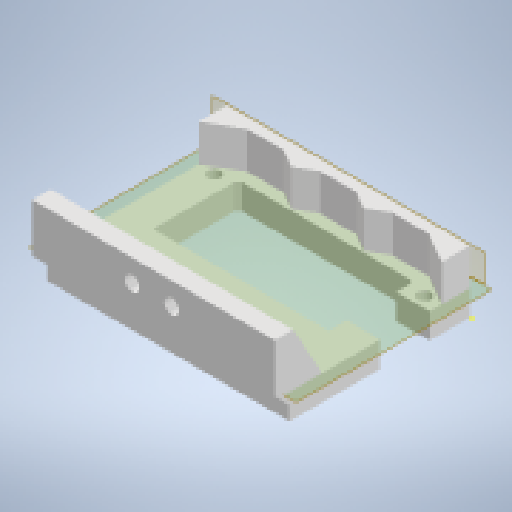
# Autodesk Inventor part: делать держит аккум
Saved by Autodesk Inventor 2024.2 (Build 282272000, 272)
## iProperties
Created: 2026-04-23
Part Number: делать держит аккум
Material: Типовые
Document SubType Name: Sheet Metal
Designer: katya_notebook
Density: 1 g/cm^3
Appearance: По умолчанию
Sheet Metal Rule: По умолчанию
Author: katya_notebook
Autodesk Inventor part; units mm, degrees
(part 1 of 2)
ref_plane "YZ Plane" through (0, 0, 0) normal (1, 0, 0) x (0, 1, 0)
ref_plane "XZ Plane" through (0, 0, 0) normal (0, 1, 0) x (-1, 0, 0)
ref_plane "XY Plane" through (0, 0, 0) normal (0, 0, 1) x (1, 0, 0)
ref_plane "РабПлоскость1" through (0, 0, 0) normal (0, 0, 1) x (1, 0, 0)
sketch "Эскиз1" plane through (0, 0, 0) normal (0, 0, 1) x (1, 0, 0)
  line L0 (-67, 0) -> (-67, 6.8113) projected
  line L1 (-67, 6.8113) -> (-59, 6.8113)
  line L2 (-59, 6.8113) -> (-59, 0)
  line L3 (-59, 0) -> (-67, 0)
  line L4 (-67, 0) -> (-67, 6.8113)
  line L5 (0, 6.8113) -> (0, 0) projected
  line L6 (0, 0) -> (-8, 0)
  line L7 (-8, 0) -> (-8, 6.8113)
  line L8 (-8, 6.8113) -> (0, 6.8113)
  line L9 (0, 6.8113) -> (0, 0)
  circle A0 centre (-62.5001, 3.4873) radius 2.1 projected
  circle A1 centre (-4.4999, 3.4873) radius 2.1 projected
  dimension "d0" = 8
  dimension "d1" = 8
  constraints: 16 end point, 4 parallel, 2 horizontal, 2 perpendicular
  measures "d0" distance of L0.end L1.end
  measures "d1" distance of L7.end L8.end
extrude "Выдавливание1" add sketch "Эскиз1" along normal blind 3
sketch "Эскиз2" plane through (-8, 0, 0) normal (0, -1, 0) x (1, 0, 0)
  line L0 (-49.3908, 28.0506) -> (-48.3929, 29.0527) projected
  line L1 (-48.3929, 29.0527) -> (-2.693, 29.1496) projected
  line L2 (-2.693, 29.1496) -> (-1.6909, 28.1517) projected
  line L3 (-1.6909, 28.1517) -> (-1.6464, 7.1518) projected
  line L4 (-1.6464, 7.1518) -> (-2.6442, 6.1496) projected
  line L5 (-2.6442, 6.1496) -> (-48.3441, 6.0528) projected
  line L6 (-48.3441, 6.0528) -> (-49.3463, 7.0507) projected
  line L7 (-49.3463, 7.0507) -> (-49.3908, 28.0506) projected
  line L8 (-48.6136, 30.0985) -> (-51.1395, 27.2282) projected
  line L9 (-51.1395, 27.2282) -> (-54.9179, 25.0466) projected
  line L10 (-54.9179, 25.0466) -> (-58.4036, 23.0363) projected
  line L11 (-58.4036, 23.0363) -> (-58.4, 21.3316) projected
  line L12 (-58.4, 21.3316) -> (-58.4, 9.3834) projected
  line L13 (-58.4, 9.3834) -> (-58.3964, 7.6788) projected
  line L14 (-58.3964, 7.6788) -> (-54.9179, 5.6684) projected
  line L15 (-54.9179, 5.6684) -> (-45.1, 0) projected
  line L16 (-45.1, 0) -> (-35.296, 5.6604) projected
  line L17 (-35.296, 5.6604) -> (-25.4498, 0.0035) projected
  line L18 (-25.4498, 0.0035) -> (-22.0179, 2.0104) projected
  line L19 (-22.0179, 2.0104) -> (-15.7, 5.658) projected
  line L20 (-15.7, 5.658) -> (-5.9, 0) projected
  line L21 (-5.9, 0) -> (3.9179, 5.6684) projected
  line L22 (3.9179, 5.6684) -> (7.4036, 7.6788) projected
  line L23 (7.4036, 7.6788) -> (7.4, 9.3834) projected
  line L24 (7.4, 9.3834) -> (7.4, 21.3316) projected
  line L25 (7.4, 21.3316) -> (7.3964, 23.0363) projected
  line L26 (7.3964, 23.0363) -> (3.9179, 25.0466) projected
  line L27 (3.9179, 25.0466) -> (-0.048, 27.3364) projected
  line L28 (-0.048, 27.3364) -> (-2.4, 30.1965) projected
  line L29 (-2.4, 30.1965) -> (-2.4, 38.3057) projected
  line L30 (-2.4, 38.3057) -> (-2.4036, 40.0104) projected
  line L31 (-2.4036, 40.0104) -> (-5.8821, 42.0207) projected
  line L32 (-5.8821, 42.0207) -> (-15.7, 47.6891) projected
  line L33 (-15.7, 47.6891) -> (-15.7258, 47.6742) projected
  line L34 (-15.7258, 47.6742) -> (-15.7517, 47.6891) projected
  line L35 (-15.7517, 47.6891) -> (-35.3517, 47.6891) projected
  line L36 (-35.3517, 47.6891) -> (-48.6347, 40.0202) projected
  line L37 (-48.6347, 40.0202) -> (-48.6136, 30.0985) projected
  line L38 (8, 0) -> (8, 3) projected
  line L39 (0, 0) -> (0, 3) projected
  line L40 (-51, 0) -> (-51, 3) projected
  line L41 (-59, 0) -> (-59, 3) projected
  line L42 (8, 3) -> (8, 8.0252)
  line L43 (8, 8.0252) -> (8, 8.0252)
  line L44 (-59, 3) -> (-51, 3) projected
  line L45 (-51, 3) -> (-51, 3.4064)
  line L46 (-59, 3) -> (-59, 8.0252)
  line L47 (-59, 8.0252) -> (-51, 3.4064)
  line L48 (0, 3) -> (0, 3.4064)
  line L49 (8, 8.0252) -> (0, 3.4064)
  line L50 (0, 3) -> (8, 3) projected
  line L51 (0, 0) -> (-51, 0)
  line L52 (1.4001, 3) -> (1.4001, 0) projected
  circle A0 centre (-54, 8) radius 2.1 projected
  circle A1 centre (3, 8) radius 2.1 projected
  point P0 (7.4036, 7.6808)
  point P1 (-5.9, 0)
  point P2 (-5.9, 0)
  point P3 (-45.1, 0)
  point P4 (-45.1, 0)
  constraints: 16 end point, 4 point on line, 2 parallel, 2 vertical, 1 collinear, 1 perpendicular
extrude "Выдавливание2" add sketch "Эскиз2" against normal up to surface (6.8113 mm away) contours L14 L15 L45 L44 L46 L47 | L15 L51 L40 L45 | L16 L17 L18 L19 L20 L51 | L21 L48 L39 L51 | L21 L22 L49 L42 L50 L48
sketch "Эскиз3" plane through (-13.9, 0, 0) normal (0, -1, 0) x (1, 0, 0)
  line L0 (0, 0) -> (13.9, 0) projected
  line L1 (13.9, 0) -> (13.9, 8.0252) projected
  line L2 (13.9, 8.0252) -> (13.3036, 7.6808) projected
  line L3 (13.3036, 7.6808) -> (13.3036, 7.6788) projected
  line L4 (13.3036, 7.6788) -> (9.8179, 5.6684) projected
  line L5 (9.8179, 5.6684) -> (0, 0) projected
  line L6 (-16.1179, 2.0104) -> (-19.5498, 0.0035) projected
  line L7 (-19.5498, 0.0035) -> (-29.396, 5.6604) projected
  line L8 (-29.396, 5.6604) -> (-39.2, 0) projected
  line L9 (-39.2, 0) -> (0, 0) projected
  line L10 (0, 0) -> (-9.8, 5.658) projected
  line L11 (-9.8, 5.658) -> (-16.1179, 2.0104) projected
  line L12 (-53.1, 0) -> (-39.2, 0) projected
  line L13 (-39.2, 0) -> (-53.1, 8.0252) projected
  line L14 (-53.1, 0) -> (-53.1, 8.0252) projected
  point P0 (13.9, 0)
ref_plane "РабПлоскость2" through (-66.4944, -3.1253, -0.1297) normal (0, -1, 0) x (0.9999978, 0, 0.0021189)
extrude "Выдавливание3" add sketch "Эскиз3" along normal blind 10
ref_plane "РабПлоскость3" through (-33.518, -3.1253, 23.8341) normal (0, -1, 0) x (0.9999978, 0, 0.0021189)
sketch "Эскиз4" plane through (-33.518, -3.1253, 23.8341) normal (0, -1, 0) x (0.9999978, 0, 0.0021189)
  line L0 (-23.8638, 4.267) -> (-22.8638, 5.267) projected
  line L1 (-22.8638, 5.267) -> (22.8362, 5.2671) projected
  line L2 (22.8362, 5.2671) -> (23.8362, 4.2671) projected
  line L3 (23.8362, 4.2671) -> (23.8362, -16.7329) projected
  line L4 (23.8362, -16.7329) -> (22.8362, -17.7329) projected
  line L5 (22.8362, -17.7329) -> (-22.8638, -17.733) projected
  line L6 (-22.8638, -17.733) -> (-23.8638, -16.733) projected
  line L7 (-23.8638, -16.733) -> (-23.8638, 4.267) projected
  line L8 (-23.0824, 6.3133) -> (-25.6142, 3.4483) projected
  line L9 (-25.6142, 3.4483) -> (-29.3974, 1.2748) projected
  line L10 (-29.3974, 1.2748) -> (-32.8873, -0.7282) projected
  line L11 (-32.8873, -0.7282) -> (-32.8873, -2.4329) projected
  line L12 (-32.8873, -2.4329) -> (-32.9126, -14.381) projected
  line L13 (-32.9126, -14.381) -> (-32.9126, -16.0857) projected
  line L14 (-32.9126, -16.0857) -> (-29.4384, -18.1034) projected
  line L15 (-29.4384, -18.1034) -> (-19.6325, -23.7926) projected
  line L16 (-19.6325, -23.7926) -> (-9.8165, -18.153) projected
  line L17 (-9.8165, -18.153) -> (0.0176, -23.8308) projected
  line L18 (0.0176, -23.8308) -> (3.4538, -21.8311) projected
  line L19 (3.4538, -21.8311) -> (9.7794, -18.1969) projected
  line L20 (9.7794, -18.1969) -> (19.5674, -23.8757) projected
  line L21 (19.5674, -23.8757) -> (29.3974, -18.2281) projected
  line L22 (29.3974, -18.2281) -> (32.8873, -16.2251) projected
  line L23 (32.8873, -16.2251) -> (32.8873, -14.5204) projected
  line L24 (32.8873, -14.5204) -> (32.9126, -2.5723) projected
  line L25 (32.9126, -2.5723) -> (32.9126, -0.8676) projected
  line L26 (32.9126, -0.8676) -> (29.4384, 1.1501) projected
  line L27 (29.4384, 1.1501) -> (25.4773, 3.4483) projected
  line L28 (25.4773, 3.4483) -> (23.1314, 6.3133) projected
  line L29 (23.1314, 6.3133) -> (23.1486, 14.4226) projected
  line L30 (23.1486, 14.4226) -> (23.1486, 16.1272) projected
  line L31 (23.1486, 16.1272) -> (19.6744, 18.1449) projected
  line L32 (19.6744, 18.1449) -> (9.8685, 23.8341) projected
  line L33 (9.8685, 23.8341) -> (9.8426, 23.8193) projected
  line L34 (9.8426, 23.8193) -> (9.8168, 23.8342) projected
  line L35 (9.8168, 23.8342) -> (-9.7831, 23.8758) projected
  line L36 (-9.7831, 23.8758) -> (-23.0824, 16.235) projected
  line L37 (-23.0824, 16.235) -> (-23.0824, 6.3133) projected
  line L38 (32.8916, -12.4579) -> (23.8362, -12.4579)
  line L39 (-23.8638, -12.4579) -> (-32.9085, -12.4579)
  circle A0 centre (-28.5155, -15.7738) radius 2.1 projected
  circle A1 centre (28.4843, -15.8945) radius 2.1 projected
  point P0 (33.4674, -23.9051)
  constraints: 6 point on line, 4 end point, 1 perpendicular
extrude "Выдавливание4" add sketch "Эскиз4" along normal up to surface (6.8747 mm away) contours L7 L6 L5 L4 L3 L38 L24 L23 L22 L21 L20 L19 L18 L17 L16 L15 L14 L13 L12 L39 | A0 | A1
sketch "Эскиз6" plane through (-67, 6.8113, 0) normal (0, 1, 0) x (1, 0, 0)
  line L0 (62.9179, -5.6684) -> (53.1, 0) projected
  line L1 (58.009, -2.8342) -> (0, -2.8342)
  line L2 (0, 0) -> (0, -8.0252) projected
  line L3 (58.009, -2.8342) -> (67, -2.8342)
  line L4 (67, -2.8342) -> (67, 0)
  line L5 (67, 0) -> (0, 0)
  constraints: 8 end point, 2 perpendicular, 2 point on line, 1 horizontal, 1 midpoint
ref_plane "РабПлоскость4" through (-66.4944, 1.8747, -0.1297) normal (0, 1, 0) x (-0.0021189, 0, 0.9999978)
extrude "Выдавливание6" add sketch "Эскиз6" against normal blind 12.687
sketch "Эскиз5" plane through (-13.9, -10, 0) normal (0, -1, 0) x (1, 0, 0)
  circle A0 centre (8.9, 8) radius 1.75
  line L0 (13.9, 0) -> (13.9, 8.0252) projected
  line L1 (-53.1, 0) -> (13.9, 0) projected
  circle A1 centre (-48.1, 8) radius 1.75
  line L2 (-53.1, 8.0252) -> (-53.1, 0) projected
  dimension "d10" = 3.5
  dimension "d11" = 5
  dimension "d12" = 8
  dimension "d13" = 5
  dimension "d14" = 8
  constraints: 2 centre point, 1 equal radius
  measures "d10" diameter of A0
  measures "d11" distance from line of L0 A0.centre
  measures "d12" distance from line of L1 A0.centre
  measures "d13" distance from line of L2 A1.centre
  measures "d14" distance from line of L1 A1.centre
extrude "Выдавливание5" cut sketch "Эскиз5" against normal blind 20
sketch "Эскиз7" plane through (-57.3553, -10, 11.3257) normal (-0.0021195, 0, 0.9999978) x (0.9999978, 0, 0.0021195)
  line L0 (-9.0447, 0) -> (0, 0) projected
  line L1 (0, 6.8747) -> (0, 0) projected
  line L2 (0, 6.8747) -> (-9.0447, 6.8747) projected
  line L3 (-9.0447, 6.8747) -> (-9.0447, 0) projected
  line L4 (47.7, 0) -> (56.7554, 0) projected
  line L5 (56.7554, 6.8747) -> (56.7554, 0) projected
  line L6 (56.7554, 6.8747) -> (47.7, 6.8747) projected
  line L7 (47.7, 6.8747) -> (47.7, 0) projected
  point P0 (57.3312, 10)
ref_plane "РабПлоскость5" through (-43.3847, -3.2558, 47.6891) normal (0, 0, 1) x (1, 0, 0)
extrude "Выдавливание7" add sketch "Эскиз7" along normal up to surface surface through (-43.3847, -3.2558, 47.6891) normal (0, 0, 1)
sketch "Эскиз8" plane through (-57.3463, -10, 7.0507) normal (0.9999978, 0, 0.0021195) x (0.0021195, 0, -0.9999978)
  line L0 (0, 0) -> (-40.6386, 0) projected
  line L1 (-22, 6.8747) -> (-40.6386, 6.8747)
  line L2 (-40.6386, 6.8747) -> (-40.6386, 0)
  line L3 (-40.6386, 0) -> (-22, 0)
  line L4 (-22, 0) -> (-22, 6.8747)
  point P0 (7.1722, 10)
  point P1 (-22, 0)
  constraints: 8 end point, 2 parallel, 1 horizontal, 1 perpendicular, 1 other
extrude "Выдавливание8" add sketch "Эскиз8" along normal up to surface (56.7554 mm away)
sketch "Эскиз9" plane through (-9.6464, -10, 7.1518) normal (-0.9999978, 0, -0.0021195) x (-0.0021195, 0, 0.9999978)
  line L0 (0, 6.8747) -> (22, 6.8747) projected
  line L1 (16.1, 6.8747) -> (3.7768, 6.8747)
  line L2 (3.7768, 6.8747) -> (3.7768, -1.5969)
  line L3 (3.7768, -1.5969) -> (16.1, -1.5969)
  line L4 (16.1, -1.5969) -> (16.1, 6.8747)
  point P0 (-7.1722, 10)
  point P1 (16.1, 3.2747)
  point P2 (4.8, 3.2747)
  point P3 (3.7768, 6.8747)
  constraints: 8 end point, 2 parallel, 1 horizontal, 1 perpendicular, 1 point on line, 2 other
extrude "Выдавливание9" cut sketch "Эскиз9" against normal blind 10
sketch "Эскиз10" plane through (-13.9, -10, 0) normal (0, -1, 0) x (1, 0, 0)
  point P0 (13.9, 0)
sketch "Эскиз11" plane through (-0.6771, -10, 47.8094) normal (-0.0021195, 0, 0.9999978) x (0.9999978, 0, 0.0021195)
  line L0 (-66.4241, 0) -> (0.5757, 0) projected
  line L1 (-65.8001, 0) -> (0, 0)
  line L2 (0, 0) -> (0, 20.9416)
  line L3 (0, 20.9416) -> (-65.8001, 20.9416)
  line L4 (-65.8001, 0) -> (-65.8001, 6.8747) projected
  line L5 (-65.8001, 0) -> (-65.8001, 20.9416)
  line L6 (0, 0) -> (0, 6.8747) projected
  point P0 (0.5757, 10)
  point P1 (0, 0)
  point P2 (0, 0)
  point P3 (0, 3.4374)
  constraints: 8 end point, 2 perpendicular, 2 point on line, 1 horizontal, 1 midpoint, 1 parallel
extrude "Выдавливание10" add sketch "Эскиз11" along normal blind 5
sketch "Эскиз12" plane through (-0.6877, -10, 52.8094) normal (-0.0021195, 0, 0.9999978) x (0.9999978, 0, 0.0021195)
  circle A0 centre (-27.9736, 14.9416) radius 2
  circle A1 centre (-38.6915, 14.9416) radius 2
  line L0 (0, 20.9416) -> (-65.8001, 20.9416) projected
  line L1 (-51.6915, 74.9747) -> (-51.6915, 11.8747) projected
  line L2 (-14.9736, 74.9747) -> (-14.9736, 11.8747) projected
  ellipse E0 centre (-33.8246, 41.3131) end of major axis (-33.8246, 52.1631) minor radius 10.85 (-23.0231, 42.3378) -> (-42.6231, 47.662) ccw projected
  line L3 (-23.0231, 74.9747) -> (-23.0231, 42.3378) projected
  line L4 (-42.6231, 74.9747) -> (-23.0231, 74.9747) projected
  line L5 (-42.6231, 74.9747) -> (-42.6231, 47.662) projected
  point P0 (0.5757, 10)
  dimension "d27" = 4
  dimension "d28" = 4
  dimension "d29" = 6
  dimension "d30" = 6
  dimension "d31" = 13
  dimension "d32" = 13
  constraints: 2 centre point, 1 other
  measures "d27" diameter of A0
  measures "d28" diameter of A1
  measures "d29" distance from line of L0 A0.centre
  measures "d30" distance from line of L0 A1.centre
  measures "d31" distance from line of L2 A0.centre
  measures "d32" distance from line of L1 A1.centre
extrude "Выдавливание11" cut sketch "Эскиз12" against normal blind 10 contours A0 | A1
sketch "Эскиз13" plane through (-0.6877, -10, 52.8094) normal (-0.0021195, 0, 0.9999978) x (0.9999978, 0, 0.0021195)
  ellipse E0 centre (-48.3136, 112.4656) end of major axis (-48.3136, 105.9656) minor radius 6.5 (-48.3136, 105.9656) -> (-48.3136, 118.9656) ccw
  line L0 (-63.3135, 105.9656) -> (-48.3136, 105.9656)
  ellipse E1 centre (-63.3135, 112.4656) end of major axis (-63.3135, 118.9656) minor radius 6.5 (-63.3135, 118.9656) -> (-63.3135, 105.9656) ccw
  line L1 (-48.3136, 118.9656) -> (-63.3135, 118.9656)
  ellipse E2 centre (-9.0636, -8.8665) end of major axis (-9.0636, -11.3665) minor radius 2.5 (-11.5636, -8.8665) -> (-9.0636, -11.3665) ccw
  line L2 (-11.5636, -8.8665) -> (-11.5636, -6.3665)
  ellipse E3 centre (-9.0636, -6.3665) end of major axis (-9.0636, -8.8665) minor radius 2.5 (-9.0636, -3.8665) -> (-11.5636, -6.3665) ccw
  line L3 (-9.0636, -3.8665) -> (-6.5636, -3.8665)
  ellipse E4 centre (-6.5636, -6.3665) end of major axis (-6.5636, -3.8665) minor radius 2.5 (-4.0637, -6.3665) -> (-6.5636, -3.8665) ccw
  line L4 (-4.0637, -6.3665) -> (-4.0637, -8.8665)
  ellipse E5 centre (-6.5636, -8.8665) end of major axis (-6.5636, -6.3665) minor radius 2.5 (-6.5636, -11.3665) -> (-4.0637, -8.8665) ccw
  line L5 (-6.5636, -11.3665) -> (-9.0636, -11.3665)
  ellipse E6 centre (-21.5636, -8.8665) end of major axis (-21.5636, -11.3665) minor radius 2.5 (-24.0636, -8.8665) -> (-21.5636, -11.3665) ccw
  line L6 (-24.0636, -8.8665) -> (-24.0636, -6.3665)
  ellipse E7 centre (-21.5636, -6.3665) end of major axis (-21.5636, -8.8665) minor radius 2.5 (-21.5636, -3.8665) -> (-24.0636, -6.3665) ccw
  line L7 (-21.5636, -3.8665) -> (-19.0636, -3.8665)
  ellipse E8 centre (-19.0636, -6.3665) end of major axis (-19.0636, -3.8665) minor radius 2.5 (-16.5636, -6.3665) -> (-19.0636, -3.8665) ccw
  line L8 (-16.5636, -6.3665) -> (-16.5636, -8.8665)
  ellipse E9 centre (-19.0636, -8.8665) end of major axis (-19.0636, -6.3665) minor radius 2.5 (-19.0636, -11.3665) -> (-16.5636, -8.8665) ccw
  line L9 (-19.0636, -11.3665) -> (-21.5636, -11.3665)
  ellipse E10 centre (-34.0636, -8.8665) end of major axis (-34.0636, -11.3665) minor radius 2.5 (-36.5636, -8.8665) -> (-34.0636, -11.3665) ccw
  line L10 (-36.5636, -8.8665) -> (-36.5636, -6.3665)
  ellipse E11 centre (-34.0636, -6.3665) end of major axis (-34.0636, -8.8665) minor radius 2.5 (-34.0636, -3.8665) -> (-36.5636, -6.3665) ccw
  line L11 (-34.0636, -3.8665) -> (-31.5636, -3.8665)
  ellipse E12 centre (-31.5636, -6.3665) end of major axis (-31.5636, -3.8665) minor radius 2.5 (-29.0636, -6.3665) -> (-31.5636, -3.8665) ccw
  line L12 (-29.0636, -6.3665) -> (-29.0636, -8.8665)
  ellipse E13 centre (-31.5636, -8.8665) end of major axis (-31.5636, -6.3665) minor radius 2.5 (-31.5636, -11.3665) -> (-29.0636, -8.8665) ccw
  line L13 (-31.5636, -11.3665) -> (-34.0636, -11.3665)
  ellipse E14 centre (-46.5636, -8.8665) end of major axis (-46.5636, -11.3665) minor radius 2.5 (-49.0636, -8.8665) -> (-46.5636, -11.3665) ccw
  line L14 (-49.0636, -8.8665) -> (-49.0636, -6.3665)
  ellipse E15 centre (-46.5636, -6.3665) end of major axis (-46.5636, -8.8665) minor radius 2.5 (-46.5636, -3.8665) -> (-49.0636, -6.3665) ccw
  line L15 (-46.5636, -3.8665) -> (-44.0636, -3.8665)
  ellipse E16 centre (-44.0636, -6.3665) end of major axis (-44.0636, -3.8665) minor radius 2.5 (-41.5636, -6.3665) -> (-44.0636, -3.8665) ccw
  line L16 (-41.5636, -6.3665) -> (-41.5636, -8.8665)
  ellipse E17 centre (-44.0636, -8.8665) end of major axis (-44.0636, -6.3665) minor radius 2.5 (-44.0636, -11.3665) -> (-41.5636, -8.8665) ccw
  line L17 (-44.0636, -11.3665) -> (-46.5636, -11.3665)
  ellipse E18 centre (-59.0635, -8.8665) end of major axis (-59.0635, -11.3665) minor radius 2.5 (-61.5635, -8.8665) -> (-59.0635, -11.3665) ccw
  line L18 (-61.5635, -8.8665) -> (-61.5635, -6.3665)
  ellipse E19 centre (-59.0635, -6.3665) end of major axis (-59.0635, -8.8665) minor radius 2.5 (-59.0635, -3.8665) -> (-61.5635, -6.3665) ccw
  line L19 (-59.0635, -3.8665) -> (-56.5635, -3.8665)
  ellipse E20 centre (-56.5635, -6.3665) end of major axis (-56.5635, -3.8665) minor radius 2.5 (-54.0635, -6.3665) -> (-56.5635, -3.8665) ccw
  line L20 (-54.0635, -6.3665) -> (-54.0635, -8.8665)
  ellipse E21 centre (-56.5635, -8.8665) end of major axis (-56.5635, -6.3665) minor radius 2.5 (-56.5635, -11.3665) -> (-54.0635, -8.8665) ccw
  line L21 (-56.5635, -11.3665) -> (-59.0635, -11.3665)
  ellipse E22 centre (-9.0636, -20.5331) end of major axis (-9.0636, -23.0331) minor radius 2.5 (-11.5636, -20.5331) -> (-9.0636, -23.0331) ccw
  line L22 (-11.5636, -20.5331) -> (-11.5636, -18.0331)
  ellipse E23 centre (-9.0636, -18.0331) end of major axis (-9.0636, -20.5331) minor radius 2.5 (-9.0636, -15.5331) -> (-11.5636, -18.0331) ccw
  line L23 (-9.0636, -15.5331) -> (-6.5636, -15.5331)
  ellipse E24 centre (-6.5636, -18.0331) end of major axis (-6.5636, -15.5331) minor radius 2.5 (-4.0637, -18.0331) -> (-6.5636, -15.5331) ccw
  line L24 (-4.0637, -18.0331) -> (-4.0637, -20.5331)
  ellipse E25 centre (-6.5636, -20.5331) end of major axis (-6.5636, -18.0331) minor radius 2.5 (-6.5636, -23.0331) -> (-4.0637, -20.5331) ccw
  line L25 (-6.5636, -23.0331) -> (-9.0636, -23.0331)
  ellipse E26 centre (-21.5636, -20.5331) end of major axis (-21.5636, -23.0331) minor radius 2.5 (-24.0636, -20.5331) -> (-21.5636, -23.0331) ccw
  line L26 (-24.0636, -20.5331) -> (-24.0636, -18.0331)
  ellipse E27 centre (-21.5636, -18.0331) end of major axis (-21.5636, -20.5331) minor radius 2.5 (-21.5636, -15.5331) -> (-24.0636, -18.0331) ccw
  line L27 (-21.5636, -15.5331) -> (-19.0636, -15.5331)
  ellipse E28 centre (-19.0636, -18.0331) end of major axis (-19.0636, -15.5331) minor radius 2.5 (-16.5636, -18.0331) -> (-19.0636, -15.5331) ccw
  line L28 (-16.5636, -18.0331) -> (-16.5636, -20.5331)
  ellipse E29 centre (-19.0636, -20.5331) end of major axis (-19.0636, -18.0331) minor radius 2.5 (-19.0636, -23.0331) -> (-16.5636, -20.5331) ccw
  line L29 (-19.0636, -23.0331) -> (-21.5636, -23.0331)
  ellipse E30 centre (-34.0636, -20.5331) end of major axis (-34.0636, -23.0331) minor radius 2.5 (-36.5636, -20.5331) -> (-34.0636, -23.0331) ccw
  line L30 (-36.5636, -20.5331) -> (-36.5636, -18.0331)
  ellipse E31 centre (-34.0636, -18.0331) end of major axis (-34.0636, -20.5331) minor radius 2.5 (-34.0636, -15.5331) -> (-36.5636, -18.0331) ccw
  line L31 (-34.0636, -15.5331) -> (-31.5636, -15.5331)
  ellipse E32 centre (-31.5636, -18.0331) end of major axis (-31.5636, -15.5331) minor radius 2.5 (-29.0636, -18.0331) -> (-31.5636, -15.5331) ccw
  line L32 (-29.0636, -18.0331) -> (-29.0636, -20.5331)
  ellipse E33 centre (-31.5636, -20.5331) end of major axis (-31.5636, -18.0331) minor radius 2.5 (-31.5636, -23.0331) -> (-29.0636, -20.5331) ccw
  line L33 (-31.5636, -23.0331) -> (-34.0636, -23.0331)
  ellipse E34 centre (-46.5636, -20.5331) end of major axis (-46.5636, -23.0331) minor radius 2.5 (-49.0636, -20.5331) -> (-46.5636, -23.0331) ccw
  line L34 (-49.0636, -20.5331) -> (-49.0636, -18.0331)
  ellipse E35 centre (-46.5636, -18.0331) end of major axis (-46.5636, -20.5331) minor radius 2.5 (-46.5636, -15.5331) -> (-49.0636, -18.0331) ccw
  line L35 (-46.5636, -15.5331) -> (-44.0636, -15.5331)
  ellipse E36 centre (-44.0636, -18.0331) end of major axis (-44.0636, -15.5331) minor radius 2.5 (-41.5636, -18.0331) -> (-44.0636, -15.5331) ccw
  line L36 (-41.5636, -18.0331) -> (-41.5636, -20.5331)
  ellipse E37 centre (-44.0636, -20.5331) end of major axis (-44.0636, -18.0331) minor radius 2.5 (-44.0636, -23.0331) -> (-41.5636, -20.5331) ccw
  line L37 (-44.0636, -23.0331) -> (-46.5636, -23.0331)
  ellipse E38 centre (-59.0635, -20.5331) end of major axis (-59.0635, -23.0331) minor radius 2.5 (-61.5635, -20.5331) -> (-59.0635, -23.0331) ccw
  line L38 (-61.5635, -20.5331) -> (-61.5635, -18.0331)
  ellipse E39 centre (-59.0635, -18.0331) end of major axis (-59.0635, -20.5331) minor radius 2.5 (-59.0635, -15.5331) -> (-61.5635, -18.0331) ccw
  line L39 (-59.0635, -15.5331) -> (-56.5635, -15.5331)
  ellipse E40 centre (-56.5635, -18.0331) end of major axis (-56.5635, -15.5331) minor radius 2.5 (-54.0635, -18.0331) -> (-56.5635, -15.5331) ccw
  line L40 (-54.0635, -18.0331) -> (-54.0635, -20.5331)
  ellipse E41 centre (-56.5635, -20.5331) end of major axis (-56.5635, -18.0331) minor radius 2.5 (-56.5635, -23.0331) -> (-54.0635, -20.5331) ccw
  line L41 (-56.5635, -23.0331) -> (-59.0635, -23.0331)
  ellipse E42 centre (-9.0636, -32.1998) end of major axis (-9.0636, -34.6998) minor radius 2.5 (-11.5636, -32.1998) -> (-9.0636, -34.6998) ccw
  line L42 (-11.5636, -32.1998) -> (-11.5636, -29.6998)
  ellipse E43 centre (-9.0636, -29.6998) end of major axis (-9.0636, -32.1998) minor radius 2.5 (-9.0636, -27.1998) -> (-11.5636, -29.6998) ccw
  line L43 (-9.0636, -27.1998) -> (-6.5636, -27.1998)
  ellipse E44 centre (-6.5636, -29.6998) end of major axis (-6.5636, -27.1998) minor radius 2.5 (-4.0637, -29.6998) -> (-6.5636, -27.1998) ccw
  line L44 (-4.0637, -29.6998) -> (-4.0637, -32.1998)
  ellipse E45 centre (-6.5636, -32.1998) end of major axis (-6.5636, -29.6998) minor radius 2.5 (-6.5636, -34.6998) -> (-4.0637, -32.1998) ccw
  line L45 (-6.5636, -34.6998) -> (-9.0636, -34.6998)
  ellipse E46 centre (-21.5636, -32.1998) end of major axis (-21.5636, -34.6998) minor radius 2.5 (-24.0636, -32.1998) -> (-21.5636, -34.6998) ccw
  line L46 (-24.0636, -32.1998) -> (-24.0636, -29.6998)
  ellipse E47 centre (-21.5636, -29.6998) end of major axis (-21.5636, -32.1998) minor radius 2.5 (-21.5636, -27.1998) -> (-24.0636, -29.6998) ccw
  line L47 (-21.5636, -27.1998) -> (-19.0636, -27.1998)
  ellipse E48 centre (-19.0636, -29.6998) end of major axis (-19.0636, -27.1998) minor radius 2.5 (-16.5636, -29.6998) -> (-19.0636, -27.1998) ccw
  line L48 (-16.5636, -29.6998) -> (-16.5636, -32.1998)
  ellipse E49 centre (-19.0636, -32.1998) end of major axis (-19.0636, -29.6998) minor radius 2.5 (-19.0636, -34.6998) -> (-16.5636, -32.1998) ccw
  line L49 (-19.0636, -34.6998) -> (-21.5636, -34.6998)
  ellipse E50 centre (-34.0636, -32.1998) end of major axis (-34.0636, -34.6998) minor radius 2.5 (-36.5636, -32.1998) -> (-34.0636, -34.6998) ccw
  line L50 (-36.5636, -32.1998) -> (-36.5636, -29.6998)
  ellipse E51 centre (-34.0636, -29.6998) end of major axis (-34.0636, -32.1998) minor radius 2.5 (-34.0636, -27.1998) -> (-36.5636, -29.6998) ccw
  line L51 (-34.0636, -27.1998) -> (-31.5636, -27.1998)
  ellipse E52 centre (-31.5636, -29.6998) end of major axis (-31.5636, -27.1998) minor radius 2.5 (-29.0636, -29.6998) -> (-31.5636, -27.1998) ccw
  line L52 (-29.0636, -29.6998) -> (-29.0636, -32.1998)
  ellipse E53 centre (-31.5636, -32.1998) end of major axis (-31.5636, -29.6998) minor radius 2.5 (-31.5636, -34.6998) -> (-29.0636, -32.1998) ccw
  line L53 (-31.5636, -34.6998) -> (-34.0636, -34.6998)
  ellipse E54 centre (-46.5636, -32.1998) end of major axis (-46.5636, -34.6998) minor radius 2.5 (-49.0636, -32.1998) -> (-46.5636, -34.6998) ccw
  line L54 (-49.0636, -32.1998) -> (-49.0636, -29.6998)
  ellipse E55 centre (-46.5636, -29.6998) end of major axis (-46.5636, -32.1998) minor radius 2.5 (-46.5636, -27.1998) -> (-49.0636, -29.6998) ccw
  line L55 (-46.5636, -27.1998) -> (-44.0636, -27.1998)
  ellipse E56 centre (-44.0636, -29.6998) end of major axis (-44.0636, -27.1998) minor radius 2.5 (-41.5636, -29.6998) -> (-44.0636, -27.1998) ccw
  line L56 (-41.5636, -29.6998) -> (-41.5636, -32.1998)
  ellipse E57 centre (-44.0636, -32.1998) end of major axis (-44.0636, -29.6998) minor radius 2.5 (-44.0636, -34.6998) -> (-41.5636, -32.1998) ccw
  line L57 (-44.0636, -34.6998) -> (-46.5636, -34.6998)
  ellipse E58 centre (-59.0635, -32.1998) end of major axis (-59.0635, -34.6998) minor radius 2.5 (-61.5635, -32.1998) -> (-59.0635, -34.6998) ccw
  line L58 (-61.5635, -32.1998) -> (-61.5635, -29.6998)
  ellipse E59 centre (-59.0635, -29.6998) end of major axis (-59.0635, -32.1998) minor radius 2.5 (-59.0635, -27.1998) -> (-61.5635, -29.6998) ccw
  line L59 (-59.0635, -27.1998) -> (-56.5635, -27.1998)
  ellipse E60 centre (-56.5635, -29.6998) end of major axis (-56.5635, -27.1998) minor radius 2.5 (-54.0635, -29.6998) -> (-56.5635, -27.1998) ccw
  line L60 (-54.0635, -29.6998) -> (-54.0635, -32.1998)
  ellipse E61 centre (-56.5635, -32.1998) end of major axis (-56.5635, -29.6998) minor radius 2.5 (-56.5635, -34.6998) -> (-54.0635, -32.1998) ccw
  line L61 (-56.5635, -34.6998) -> (-59.0635, -34.6998)
  ellipse E62 centre (-9.0636, -43.8665) end of major axis (-9.0636, -46.3665) minor radius 2.5 (-11.5636, -43.8665) -> (-9.0636, -46.3665) ccw
  line L62 (-11.5636, -43.8665) -> (-11.5636, -41.3665)
  ellipse E63 centre (-9.0636, -41.3665) end of major axis (-9.0636, -43.8665) minor radius 2.5 (-9.0636, -38.8665) -> (-11.5636, -41.3665) ccw
  line L63 (-9.0636, -38.8665) -> (-6.5636, -38.8665)
  ellipse E64 centre (-6.5636, -41.3665) end of major axis (-6.5636, -38.8665) minor radius 2.5 (-4.0637, -41.3665) -> (-6.5636, -38.8665) ccw
  line L64 (-4.0637, -41.3665) -> (-4.0637, -43.8665)
  ellipse E65 centre (-6.5636, -43.8665) end of major axis (-6.5636, -41.3665) minor radius 2.5 (-6.5636, -46.3665) -> (-4.0637, -43.8665) ccw
  line L65 (-6.5636, -46.3665) -> (-9.0636, -46.3665)
  ellipse E66 centre (-21.5636, -43.8665) end of major axis (-21.5636, -46.3665) minor radius 2.5 (-24.0636, -43.8665) -> (-21.5636, -46.3665) ccw
  line L66 (-24.0636, -43.8665) -> (-24.0636, -41.3665)
  ellipse E67 centre (-21.5636, -41.3665) end of major axis (-21.5636, -43.8665) minor radius 2.5 (-21.5636, -38.8665) -> (-24.0636, -41.3665) ccw
  line L67 (-21.5636, -38.8665) -> (-19.0636, -38.8665)
  ellipse E68 centre (-19.0636, -41.3665) end of major axis (-19.0636, -38.8665) minor radius 2.5 (-16.5636, -41.3665) -> (-19.0636, -38.8665) ccw
  line L68 (-16.5636, -41.3665) -> (-16.5636, -43.8665)
  ellipse E69 centre (-19.0636, -43.8665) end of major axis (-19.0636, -41.3665) minor radius 2.5 (-19.0636, -46.3665) -> (-16.5636, -43.8665) ccw
  line L69 (-19.0636, -46.3665) -> (-21.5636, -46.3665)
  ellipse E70 centre (-34.0636, -43.8665) end of major axis (-34.0636, -46.3665) minor radius 2.5 (-36.5636, -43.8665) -> (-34.0636, -46.3665) ccw
  line L70 (-36.5636, -43.8665) -> (-36.5636, -41.3665)
  ellipse E71 centre (-34.0636, -41.3665) end of major axis (-34.0636, -43.8665) minor radius 2.5 (-34.0636, -38.8665) -> (-36.5636, -41.3665) ccw
  line L71 (-34.0636, -38.8665) -> (-31.5636, -38.8665)
  ellipse E72 centre (-31.5636, -41.3665) end of major axis (-31.5636, -38.8665) minor radius 2.5 (-29.0636, -41.3665) -> (-31.5636, -38.8665) ccw
  line L72 (-29.0636, -41.3665) -> (-29.0636, -43.8665)
  ellipse E73 centre (-31.5636, -43.8665) end of major axis (-31.5636, -41.3665) minor radius 2.5 (-31.5636, -46.3665) -> (-29.0636, -43.8665) ccw
  line L73 (-31.5636, -46.3665) -> (-34.0636, -46.3665)
  ellipse E74 centre (-46.5636, -43.8665) end of major axis (-46.5636, -46.3665) minor radius 2.5 (-49.0636, -43.8665) -> (-46.5636, -46.3665) ccw
  line L74 (-49.0636, -43.8665) -> (-49.0636, -41.3665)
  ellipse E75 centre (-46.5636, -41.3665) end of major axis (-46.5636, -43.8665) minor radius 2.5 (-46.5636, -38.8665) -> (-49.0636, -41.3665) ccw
  line L75 (-46.5636, -38.8665) -> (-44.0636, -38.8665)
  ellipse E76 centre (-44.0636, -41.3665) end of major axis (-44.0636, -38.8665) minor radius 2.5 (-41.5636, -41.3665) -> (-44.0636, -38.8665) ccw
  line L76 (-41.5636, -41.3665) -> (-41.5636, -43.8665)
  ellipse E77 centre (-44.0636, -43.8665) end of major axis (-44.0636, -41.3665) minor radius 2.5 (-44.0636, -46.3665) -> (-41.5636, -43.8665) ccw
  line L77 (-44.0636, -46.3665) -> (-46.5636, -46.3665)
  ellipse E78 centre (-59.0635, -43.8665) end of major axis (-59.0635, -46.3665) minor radius 2.5 (-61.5635, -43.8665) -> (-59.0635, -46.3665) ccw
  line L78 (-61.5635, -43.8665) -> (-61.5635, -41.3665)
  ellipse E79 centre (-59.0635, -41.3665) end of major axis (-59.0635, -43.8665) minor radius 2.5 (-59.0635, -38.8665) -> (-61.5635, -41.3665) ccw
  line L79 (-59.0635, -38.8665) -> (-56.5635, -38.8665)
  ellipse E80 centre (-56.5635, -41.3665) end of major axis (-56.5635, -38.8665) minor radius 2.5 (-54.0635, -41.3665) -> (-56.5635, -38.8665) ccw
  line L80 (-54.0635, -41.3665) -> (-54.0635, -43.8665)
  ellipse E81 centre (-56.5635, -43.8665) end of major axis (-56.5635, -41.3665) minor radius 2.5 (-56.5635, -46.3665) -> (-54.0635, -43.8665) ccw
  line L81 (-56.5635, -46.3665) -> (-59.0635, -46.3665)
  ellipse E82 centre (-9.0636, -55.5331) end of major axis (-9.0636, -58.0331) minor radius 2.5 (-11.5636, -55.5331) -> (-9.0636, -58.0331) ccw
  line L82 (-11.5636, -55.5331) -> (-11.5636, -53.0331)
  ellipse E83 centre (-9.0636, -53.0331) end of major axis (-9.0636, -55.5331) minor radius 2.5 (-9.0636, -50.5331) -> (-11.5636, -53.0331) ccw
  line L83 (-9.0636, -50.5331) -> (-6.5636, -50.5331)
  ellipse E84 centre (-6.5636, -53.0331) end of major axis (-6.5636, -50.5331) minor radius 2.5 (-4.0637, -53.0331) -> (-6.5636, -50.5331) ccw
  line L84 (-4.0637, -53.0331) -> (-4.0637, -55.5331)
  ellipse E85 centre (-6.5636, -55.5331) end of major axis (-6.5636, -53.0331) minor radius 2.5 (-6.5636, -58.0331) -> (-4.0637, -55.5331) ccw
  line L85 (-6.5636, -58.0331) -> (-9.0636, -58.0331)
  ellipse E86 centre (-21.5636, -55.5331) end of major axis (-21.5636, -58.0331) minor radius 2.5 (-24.0636, -55.5331) -> (-21.5636, -58.0331) ccw
  line L86 (-24.0636, -55.5331) -> (-24.0636, -53.0331)
  ellipse E87 centre (-21.5636, -53.0331) end of major axis (-21.5636, -55.5331) minor radius 2.5 (-21.5636, -50.5331) -> (-24.0636, -53.0331) ccw
  line L87 (-21.5636, -50.5331) -> (-19.0636, -50.5331)
  ellipse E88 centre (-19.0636, -53.0331) end of major axis (-19.0636, -50.5331) minor radius 2.5 (-16.5636, -53.0331) -> (-19.0636, -50.5331) ccw
  line L88 (-16.5636, -53.0331) -> (-16.5636, -55.5331)
  ellipse E89 centre (-19.0636, -55.5331) end of major axis (-19.0636, -53.0331) minor radius 2.5 (-19.0636, -58.0331) -> (-16.5636, -55.5331) ccw
  line L89 (-19.0636, -58.0331) -> (-21.5636, -58.0331)
  ellipse E90 centre (-34.0636, -55.5331) end of major axis (-34.0636, -58.0331) minor radius 2.5 (-36.5636, -55.5331) -> (-34.0636, -58.0331) ccw
  line L90 (-36.5636, -55.5331) -> (-36.5636, -53.0331)
  ellipse E91 centre (-34.0636, -53.0331) end of major axis (-34.0636, -55.5331) minor radius 2.5 (-34.0636, -50.5331) -> (-36.5636, -53.0331) ccw
  line L91 (-34.0636, -50.5331) -> (-31.5636, -50.5331)
  ellipse E92 centre (-31.5636, -53.0331) end of major axis (-31.5636, -50.5331) minor radius 2.5 (-29.0636, -53.0331) -> (-31.5636, -50.5331) ccw
  line L92 (-29.0636, -53.0331) -> (-29.0636, -55.5331)
  ellipse E93 centre (-31.5636, -55.5331) end of major axis (-31.5636, -53.0331) minor radius 2.5 (-31.5636, -58.0331) -> (-29.0636, -55.5331) ccw
  line L93 (-31.5636, -58.0331) -> (-34.0636, -58.0331)
  ellipse E94 centre (-46.5636, -55.5331) end of major axis (-46.5636, -58.0331) minor radius 2.5 (-49.0636, -55.5331) -> (-46.5636, -58.0331) ccw
  line L94 (-49.0636, -55.5331) -> (-49.0636, -53.0331)
  ellipse E95 centre (-46.5636, -53.0331) end of major axis (-46.5636, -55.5331) minor radius 2.5 (-46.5636, -50.5331) -> (-49.0636, -53.0331) ccw
  line L95 (-46.5636, -50.5331) -> (-44.0636, -50.5331)
  ellipse E96 centre (-44.0636, -53.0331) end of major axis (-44.0636, -50.5331) minor radius 2.5 (-41.5636, -53.0331) -> (-44.0636, -50.5331) ccw
  line L96 (-41.5636, -53.0331) -> (-41.5636, -55.5331)
  ellipse E97 centre (-44.0636, -55.5331) end of major axis (-44.0636, -53.0331) minor radius 2.5 (-44.0636, -58.0331) -> (-41.5636, -55.5331) ccw
  line L97 (-44.0636, -58.0331) -> (-46.5636, -58.0331)
  ellipse E98 centre (-59.0635, -55.5331) end of major axis (-59.0635, -58.0331) minor radius 2.5 (-61.5635, -55.5331) -> (-59.0635, -58.0331) ccw
  line L98 (-61.5635, -55.5331) -> (-61.5635, -53.0331)
  ellipse E99 centre (-59.0635, -53.0331) end of major axis (-59.0635, -55.5331) minor radius 2.5 (-59.0635, -50.5331) -> (-61.5635, -53.0331) ccw
  line L99 (-59.0635, -50.5331) -> (-56.5635, -50.5331)
  ellipse E100 centre (-56.5635, -53.0331) end of major axis (-56.5635, -50.5331) minor radius 2.5 (-54.0635, -53.0331) -> (-56.5635, -50.5331) ccw
  line L100 (-54.0635, -53.0331) -> (-54.0635, -55.5331)
  ellipse E101 centre (-56.5635, -55.5331) end of major axis (-56.5635, -53.0331) minor radius 2.5 (-56.5635, -58.0331) -> (-54.0635, -55.5331) ccw
  line L101 (-56.5635, -58.0331) -> (-59.0635, -58.0331)
  ellipse E102 centre (-9.0636, -67.1998) end of major axis (-9.0636, -69.6998) minor radius 2.5 (-11.5636, -67.1998) -> (-9.0636, -69.6998) ccw
  line L102 (-11.5636, -67.1998) -> (-11.5636, -64.6998)
  ellipse E103 centre (-9.0636, -64.6998) end of major axis (-9.0636, -67.1998) minor radius 2.5 (-9.0636, -62.1998) -> (-11.5636, -64.6998) ccw
  line L103 (-9.0636, -62.1998) -> (-6.5636, -62.1998)
  ellipse E104 centre (-6.5636, -64.6998) end of major axis (-6.5636, -62.1998) minor radius 2.5 (-4.0637, -64.6998) -> (-6.5636, -62.1998) ccw
  line L104 (-4.0637, -64.6998) -> (-4.0637, -67.1998)
  ellipse E105 centre (-6.5636, -67.1998) end of major axis (-6.5636, -64.6998) minor radius 2.5 (-6.5636, -69.6998) -> (-4.0637, -67.1998) ccw
  line L105 (-6.5636, -69.6998) -> (-9.0636, -69.6998)
  ellipse E106 centre (-21.5636, -67.1998) end of major axis (-21.5636, -69.6998) minor radius 2.5 (-24.0636, -67.1998) -> (-21.5636, -69.6998) ccw
  line L106 (-24.0636, -67.1998) -> (-24.0636, -64.6998)
  ellipse E107 centre (-21.5636, -64.6998) end of major axis (-21.5636, -67.1998) minor radius 2.5 (-21.5636, -62.1998) -> (-24.0636, -64.6998) ccw
  line L107 (-21.5636, -62.1998) -> (-19.0636, -62.1998)
  ellipse E108 centre (-19.0636, -64.6998) end of major axis (-19.0636, -62.1998) minor radius 2.5 (-16.5636, -64.6998) -> (-19.0636, -62.1998) ccw
  line L108 (-16.5636, -64.6998) -> (-16.5636, -67.1998)
  ellipse E109 centre (-19.0636, -67.1998) end of major axis (-19.0636, -64.6998) minor radius 2.5 (-19.0636, -69.6998) -> (-16.5636, -67.1998) ccw
  line L109 (-19.0636, -69.6998) -> (-21.5636, -69.6998)
  ellipse E110 centre (-34.0636, -67.1998) end of major axis (-34.0636, -69.6998) minor radius 2.5 (-36.5636, -67.1998) -> (-34.0636, -69.6998) ccw
  line L110 (-36.5636, -67.1998) -> (-36.5636, -64.6998)
  ellipse E111 centre (-34.0636, -64.6998) end of major axis (-34.0636, -67.1998) minor radius 2.5 (-34.0636, -62.1998) -> (-36.5636, -64.6998) ccw
  line L111 (-34.0636, -62.1998) -> (-31.5636, -62.1998)
  ellipse E112 centre (-31.5636, -64.6998) end of major axis (-31.5636, -62.1998) minor radius 2.5 (-29.0636, -64.6998) -> (-31.5636, -62.1998) ccw
  line L112 (-29.0636, -64.6998) -> (-29.0636, -67.1998)
  ellipse E113 centre (-31.5636, -67.1998) end of major axis (-31.5636, -64.6998) minor radius 2.5 (-31.5636, -69.6998) -> (-29.0636, -67.1998) ccw
  line L113 (-31.5636, -69.6998) -> (-34.0636, -69.6998)
  ellipse E114 centre (-46.5636, -67.1998) end of major axis (-46.5636, -69.6998) minor radius 2.5 (-49.0636, -67.1998) -> (-46.5636, -69.6998) ccw
  line L114 (-49.0636, -67.1998) -> (-49.0636, -64.6998)
  ellipse E115 centre (-46.5636, -64.6998) end of major axis (-46.5636, -67.1998) minor radius 2.5 (-46.5636, -62.1998) -> (-49.0636, -64.6998) ccw
  line L115 (-46.5636, -62.1998) -> (-44.0636, -62.1998)
  ellipse E116 centre (-44.0636, -64.6998) end of major axis (-44.0636, -62.1998) minor radius 2.5 (-41.5636, -64.6998) -> (-44.0636, -62.1998) ccw
  line L116 (-41.5636, -64.6998) -> (-41.5636, -67.1998)
  ellipse E117 centre (-44.0636, -67.1998) end of major axis (-44.0636, -64.6998) minor radius 2.5 (-44.0636, -69.6998) -> (-41.5636, -67.1998) ccw
  line L117 (-44.0636, -69.6998) -> (-46.5636, -69.6998)
  ellipse E118 centre (-9.0636, -78.8665) end of major axis (-9.0636, -81.3665) minor radius 2.5 (-11.5636, -78.8665) -> (-9.0636, -81.3665) ccw
  line L118 (-11.5636, -78.8665) -> (-11.5636, -76.3665)
  ellipse E119 centre (-9.0636, -76.3665) end of major axis (-9.0636, -78.8665) minor radius 2.5 (-9.0636, -73.8665) -> (-11.5636, -76.3665) ccw
  line L119 (-9.0636, -73.8665) -> (-6.5636, -73.8665)
  ellipse E120 centre (-6.5636, -76.3665) end of major axis (-6.5636, -73.8665) minor radius 2.5 (-4.0637, -76.3665) -> (-6.5636, -73.8665) ccw
  line L120 (-4.0637, -76.3665) -> (-4.0637, -78.8665)
  ellipse E121 centre (-6.5636, -78.8665) end of major axis (-6.5636, -76.3665) minor radius 2.5 (-6.5636, -81.3665) -> (-4.0637, -78.8665) ccw
  line L121 (-6.5636, -81.3665) -> (-9.0636, -81.3665)
  ellipse E122 centre (-21.5636, -78.8665) end of major axis (-21.5636, -81.3665) minor radius 2.5 (-24.0636, -78.8665) -> (-21.5636, -81.3665) ccw
  line L122 (-24.0636, -78.8665) -> (-24.0636, -76.3665)
  ellipse E123 centre (-21.5636, -76.3665) end of major axis (-21.5636, -78.8665) minor radius 2.5 (-21.5636, -73.8665) -> (-24.0636, -76.3665) ccw
  line L123 (-21.5636, -73.8665) -> (-19.0636, -73.8665)
  ellipse E124 centre (-19.0636, -76.3665) end of major axis (-19.0636, -73.8665) minor radius 2.5 (-16.5636, -76.3665) -> (-19.0636, -73.8665) ccw
  line L124 (-16.5636, -76.3665) -> (-16.5636, -78.8665)
  ellipse E125 centre (-19.0636, -78.8665) end of major axis (-19.0636, -76.3665) minor radius 2.5 (-19.0636, -81.3665) -> (-16.5636, -78.8665) ccw
  line L125 (-19.0636, -81.3665) -> (-21.5636, -81.3665)
  ellipse E126 centre (-34.0636, -78.8665) end of major axis (-34.0636, -81.3665) minor radius 2.5 (-36.5636, -78.8665) -> (-34.0636, -81.3665) ccw
  line L126 (-36.5636, -78.8665) -> (-36.5636, -76.3665)
  ellipse E127 centre (-34.0636, -76.3665) end of major axis (-34.0636, -78.8665) minor radius 2.5 (-34.0636, -73.8665) -> (-36.5636, -76.3665) ccw
  line L127 (-34.0636, -73.8665) -> (-31.5636, -73.8665)
  ellipse E128 centre (-31.5636, -76.3665) end of major axis (-31.5636, -73.8665) minor radius 2.5 (-29.0636, -76.3665) -> (-31.5636, -73.8665) ccw
  line L128 (-29.0636, -76.3665) -> (-29.0636, -78.8665)
  ellipse E129 centre (-31.5636, -78.8665) end of major axis (-31.5636, -76.3665) minor radius 2.5 (-31.5636, -81.3665) -> (-29.0636, -78.8665) ccw
  line L129 (-31.5636, -81.3665) -> (-34.0636, -81.3665)
  ellipse E130 centre (-46.5636, -78.8665) end of major axis (-46.5636, -81.3665) minor radius 2.5 (-49.0636, -78.8665) -> (-46.5636, -81.3665) ccw
  line L130 (-49.0636, -78.8665) -> (-49.0636, -76.3665)
  ellipse E131 centre (-46.5636, -76.3665) end of major axis (-46.5636, -78.8665) minor radius 2.5 (-46.5636, -73.8665) -> (-49.0636, -76.3665) ccw
  line L131 (-46.5636, -73.8665) -> (-44.0636, -73.8665)
  ellipse E132 centre (-44.0636, -76.3665) end of major axis (-44.0636, -73.8665) minor radius 2.5 (-41.5636, -76.3665) -> (-44.0636, -73.8665) ccw
  line L132 (-41.5636, -76.3665) -> (-41.5636, -78.8665)
  ellipse E133 centre (-44.0636, -78.8665) end of major axis (-44.0636, -76.3665) minor radius 2.5 (-44.0636, -81.3665) -> (-41.5636, -78.8665) ccw
  line L133 (-44.0636, -81.3665) -> (-46.5636, -81.3665)
  line L134 (-56.5635, -69.6998) -> (-59.0635, -69.6998)
  ellipse E134 centre (-59.0635, -67.1998) end of major axis (-59.0635, -69.6998) minor radius 2.5 (-61.5635, -67.1998) -> (-59.0635, -69.6998) ccw
  line L135 (-61.5635, -67.1998) -> (-61.5635, -64.6998)
  ellipse E135 centre (-59.0635, -64.6998) end of major axis (-59.0635, -67.1998) minor radius 2.5 (-59.0635, -62.1998) -> (-61.5635, -64.6998) ccw
  line L136 (-59.0635, -62.1998) -> (-56.5635, -62.1998)
  ellipse E136 centre (-56.5635, -64.6998) end of major axis (-56.5635, -62.1998) minor radius 2.5 (-54.0635, -64.6998) -> (-56.5635, -62.1998) ccw
  line L137 (-54.0635, -64.6998) -> (-54.0635, -67.1998)
  ellipse E137 centre (-56.5635, -67.1998) end of major axis (-56.5635, -64.6998) minor radius 2.5 (-56.5635, -69.6998) -> (-54.0635, -67.1998) ccw
  line L138 (-66.3135, 5.3835) -> (-66.3135, 102.6157)
  line L139 (-66.3135, 102.6157) -> (0.6863, 102.6157)
  line L140 (0.6863, 102.6157) -> (0.6863, 5.3835)
  line L141 (0.6863, 5.3835) -> (-66.3135, 5.3835)
  ellipse E138 centre (-17.3136, 112.4656) end of major axis (-17.3136, 118.9656) minor radius 6.5 (-17.3136, 118.9656) -> (-17.3136, 105.9656) ccw
  line L142 (-2.3137, 118.9656) -> (-17.3136, 118.9656)
  ellipse E139 centre (-2.3137, 112.4656) end of major axis (-2.3137, 105.9656) minor radius 6.5 (-2.3137, 105.9656) -> (-2.3137, 118.9656) ccw
  line L143 (-17.3136, 105.9656) -> (-2.3137, 105.9656)
  ellipse E140 centre (-59.0635, -78.8665) end of major axis (-59.0635, -81.3665) minor radius 2.5 (-61.5635, -78.8665) -> (-59.0635, -81.3665) ccw
  line L144 (-61.5635, -78.8665) -> (-61.5635, -76.3665)
  ellipse E141 centre (-59.0635, -76.3665) end of major axis (-59.0635, -78.8665) minor radius 2.5 (-59.0635, -73.8665) -> (-61.5635, -76.3665) ccw
  line L145 (-59.0635, -73.8665) -> (-56.5635, -73.8665)
  ellipse E142 centre (-56.5635, -76.3665) end of major axis (-56.5635, -73.8665) minor radius 2.5 (-54.0635, -76.3665) -> (-56.5635, -73.8665) ccw
  line L146 (-54.0635, -76.3665) -> (-54.0635, -78.8665)
  ellipse E143 centre (-56.5635, -78.8665) end of major axis (-56.5635, -76.3665) minor radius 2.5 (-56.5635, -81.3665) -> (-54.0635, -78.8665) ccw
  line L147 (-56.5635, -81.3665) -> (-59.0635, -81.3665)
  line L148 (7.5063, -92.7382) -> (7.5063, -83.9202)
  line L149 (10.7063, -83.9202) -> (7.5063, -83.9202)
  line L150 (10.7063, -55.6448) -> (10.7063, -83.9202)
  line L151 (10.7063, -54.6448) -> (10.7063, -55.6448)
  spline S0 degree 3 poles (13.7063, -50.8164) (13.1746, -50.8164) (12.6519, -51.0007) (11.9339, -51.513) (11.6833, -51.7737) (11.4756, -52.0675) (11.2679, -52.3612) (11.1024, -52.6885) (10.7973, -53.5437) (10.7063, -54.0942) (10.7063, -54.6448) knots 0 0 0 0 0.4672 0.4672 0.785398 0.785398 0.785398 1.103596 1.103596 1.570796 1.570796 1.570796 1.570796 weights 1 1 1 1 1 1 1 1 1 1 1
  line L152 (17.1863, -50.8164) -> (13.7063, -50.8164)
  line L153 (17.1863, -24.2525) -> (17.1863, -50.8164)
  line L154 (7.4097, -24.2525) -> (17.1863, -24.2525)
  spline S1 degree 3 poles (5.179, -23.0014) (5.2766, -23.1394) (5.3836, -23.2701) (5.6889, -23.5888) (5.9029, -23.7618) (6.1389, -23.9001) (6.3295, -24.0117) (6.5346, -24.1005) (6.963, -24.2211) (7.1863, -24.2525) (7.4097, -24.2525) knots -0.785398 -0.785398 -0.785398 -0.785398 -0.635897 -0.635897 -0.392699 -0.392699 -0.392699 -0.19635 -0.19635 0 0 0 0 weights 1 1 1 1 1 1 1 1 1 1 1
  line L155 (4.7708, -22.4241) -> (5.179, -23.0014)
  line L156 (2.7756, -19.6025) -> (4.7708, -22.4241)
  spline S2 degree 3 poles (2.2549, -18.5661) (2.3178, -18.7521) (2.3926, -18.9329) (2.5662, -19.2797) (2.6649, -19.4459) (2.7756, -19.6025) knots 0 0 0 0 0.5 0.5 1 1 1 1 weights 1 1 1 1 1 1
  spline S3 degree 3 poles (2.0063, -17.0251) (2.0063, -17.052) (2.0065, -17.079) (2.014, -17.5417) (2.0781, -17.9762) (2.1989, -18.3886) (2.2164, -18.4483) (2.235, -18.5075) (2.2549, -18.5661) knots 0 0 0 0 0.051197 0.051197 0.880094 0.880094 0.880094 1 1 1 1 weights 1 1 1 1 1 1 1 1 1
  line L157 (2.0063, -16.0251) -> (2.0063, -17.0251)
  line L158 (2.0063, 94.3552) -> (2.0063, -16.0251)
  line L159 (2.0063, 95.3552) -> (2.0063, 94.3552)
  spline S4 degree 3 poles (5.0063, 99.1836) (4.4746, 99.1836) (3.9519, 98.9993) (3.2339, 98.487) (2.9834, 98.2263) (2.7756, 97.9325) (2.5679, 97.6388) (2.4024, 97.3115) (2.0973, 96.4563) (2.0063, 95.9058) (2.0063, 95.3552) knots 0 0 0 0 0.4672 0.4672 0.785398 0.785398 0.785398 1.103596 1.103596 1.570796 1.570796 1.570796 1.570796 weights 1 1 1 1 1 1 1 1 1 1 1
  line L160 (6.1863, 99.1836) -> (5.0063, 99.1836)
  line L161 (6.1863, 125.7475) -> (6.1863, 99.1836)
  line L162 (-71.8135, 125.7475) -> (6.1863, 125.7475)
  line L163 (-71.8135, 99.1836) -> (-71.8135, 125.7475)
  line L164 (-70.6335, 99.1836) -> (-71.8135, 99.1836)
  spline S5 degree 3 poles (-67.6335, 95.3552) (-67.6335, 95.9058) (-67.7245, 96.4563) (-68.0296, 97.3115) (-68.1951, 97.6388) (-68.4028, 97.9325) (-68.6105, 98.2263) (-68.8611, 98.487) (-69.5791, 98.9993) (-70.1018, 99.1836) (-70.6335, 99.1836) knots -1.570796 -1.570796 -1.570796 -1.570796 -1.103596 -1.103596 -0.785398 -0.785398 -0.785398 -0.4672 -0.4672 0 0 0 0 weights 1 1 1 1 1 1 1 1 1 1 1
  line L165 (-67.6335, 94.3552) -> (-67.6335, 95.3552)
  line L166 (-67.6335, -16.0251) -> (-67.6335, 94.3552)
  line L167 (-67.6335, -17.0251) -> (-67.6335, -16.0251)
  spline S6 degree 3 poles (-67.8821, -18.5661) (-67.8622, -18.5075) (-67.8435, -18.4483) (-67.8261, -18.3886) (-67.7053, -17.9762) (-67.6412, -17.5417) (-67.6337, -17.079) (-67.6335, -17.052) (-67.6335, -17.0251) knots 0 0 0 0 0.119906 0.119906 0.119906 0.948803 0.948803 1 1 1 1 weights 1 1 1 1 1 1 1 1 1
  spline S7 degree 3 poles (-68.4028, -19.6025) (-68.2921, -19.4459) (-68.1934, -19.2797) (-68.0198, -18.9329) (-67.945, -18.7521) (-67.8821, -18.5661) knots 0 0 0 0 0.5 0.5 1 1 1 1 weights 1 1 1 1 1 1
  line L168 (-70.398, -22.4241) -> (-68.4028, -19.6025)
  line L169 (-70.8062, -23.0014) -> (-70.398, -22.4241)
  spline S8 degree 3 poles (-73.0369, -24.2525) (-72.8135, -24.2525) (-72.5902, -24.2211) (-72.1617, -24.1005) (-71.9567, -24.0117) (-71.7661, -23.9001) (-71.53, -23.7618) (-71.3161, -23.5888) (-71.0108, -23.2701) (-70.9038, -23.1394) (-70.8062, -23.0014) knots 0 0 0 0 0.19635 0.19635 0.392699 0.392699 0.392699 0.635897 0.635897 0.785398 0.785398 0.785398 0.785398 weights 1 1 1 1 1 1 1 1 1 1 1
  line L170 (-82.8135, -24.2525) -> (-73.0369, -24.2525)
  line L171 (-82.8135, -50.8164) -> (-82.8135, -24.2525)
  line L172 (-79.3335, -50.8164) -> (-82.8135, -50.8164)
  spline S9 degree 3 poles (-76.3335, -54.6448) (-76.3335, -54.0942) (-76.4245, -53.5437) (-76.7295, -52.6885) (-76.895, -52.3612) (-77.1028, -52.0675) (-77.3105, -51.7737) (-77.561, -51.513) (-78.2791, -51.0007) (-78.8018, -50.8164) (-79.3335, -50.8164) knots -1.570796 -1.570796 -1.570796 -1.570796 -1.103596 -1.103596 -0.785398 -0.785398 -0.785398 -0.4672 -0.4672 0 0 0 0 weights 1 1 1 1 1 1 1 1 1 1 1
  line L173 (-76.3335, -55.6448) -> (-76.3335, -54.6448)
  line L174 (-76.3335, -83.9202) -> (-76.3335, -55.6448)
  line L175 (-73.1335, -83.9202) -> (-76.3335, -83.9202)
  line L176 (-73.1335, -83.9202) -> (-73.1335, -92.7382)
  line L177 (-69.8103, -92.7382) -> (-73.1335, -92.7382)
  ellipse E144 centre (-63.3135, -92.5344) end of major axis (-63.3135, -86.0344) minor radius 6.5 (-63.3135, -86.0344) -> (-69.8103, -92.7382) ccw
  line L178 (-48.3136, -86.0344) -> (-63.3135, -86.0344)
  ellipse E145 centre (-48.3136, -92.5344) end of major axis (-48.3136, -99.0344) minor radius 6.5 (-41.8168, -92.7382) -> (-48.3136, -86.0344) ccw
  line L179 (-23.8104, -92.7382) -> (-41.8168, -92.7382)
  ellipse E146 centre (-17.3136, -92.5344) end of major axis (-17.3136, -86.0344) minor radius 6.5 (-17.3136, -86.0344) -> (-23.8104, -92.7382) ccw
  line L180 (-2.3137, -86.0344) -> (-17.3136, -86.0344)
  ellipse E147 centre (-2.3137, -92.5344) end of major axis (-2.3137, -99.0344) minor radius 6.5 (4.1831, -92.7382) -> (-2.3137, -86.0344) ccw
  line L181 (7.5063, -92.7382) -> (4.1831, -92.7382)
  line L182 (0.6863, 7.763) -> (-67.6335, 7.763)
  line L183 (-67.6335, 7.763) -> (-67.6335, 0)
  line L184 (-67.6335, 0) -> (0.6863, 0)
  line L185 (0.6863, 0) -> (0.6863, 7.763)
  point P0 (0.5757, 10)
  point P1 (0.6863, 5.3835)
  point P2 (-67.6335, 7.763)
  constraints: 8 end point, 2 parallel, 2 point on line, 1 horizontal, 1 perpendicular, 148 other
extrude "Выдавливание12" cut sketch "Эскиз13" against normal blind 4 contours L141 L185 L184 L166 L182 L138 | L138 L182 L140 L141
sketch "Эскиз14" plane through (-13.9, -10, 0) normal (0, -1, 0) x (1, 0, 0)
  line L0 (13.9, 0) -> (13.9, 8.0252) projected
  line L1 (13.3, 9.3834) -> (13.3036, 7.6808) projected
  line L2 (13.9, 0) -> (13.3011, 0)
  line L3 (13.3011, 0) -> (13.3011, 8.8822)
  line L4 (13.3011, 8.8822) -> (13.9, 8.8822)
  line L5 (13.9, 8.8822) -> (13.9, 0)
  line L6 (-53.1, 0) -> (13.9, 0) projected
  line L7 (-52.5, 9.3834) -> (-52.5, 11.3065) projected
  line L8 (-53.1, 0) -> (-52.5, 0)
  line L9 (-52.5, 0) -> (-52.5, 9.3834)
  line L10 (-52.5, 9.3834) -> (-53.1, 9.3834)
  line L11 (-53.1, 9.3834) -> (-53.1, 0)
  constraints: 16 end point, 4 parallel, 2 horizontal, 2 perpendicular, 1 point on line
extrude "Выдавливание13" cut sketch "Эскиз14" against normal up to surface (16.8113 mm away)
sketch "Эскиз15" plane through (-9.6805, -10, 23.2517) normal (0.0021195, 0, -0.9999978) x (-0.9999978, 0, -0.0021195)
  line L0 (-9.0554, 6.8747) -> (0, 6.8747) projected
  line L1 (0, 0) -> (-9.0554, 0) projected
  line L2 (0, 6.8747) -> (0, 0) projected
  line L3 (-9.0554, 6.8747) -> (0, 6.8747) projected
  line L4 (-9.0554, 0) -> (-9.0554, 6.8747) projected
  point P0 (-9.6312, 10)
  point P1 (0, 6.8747)